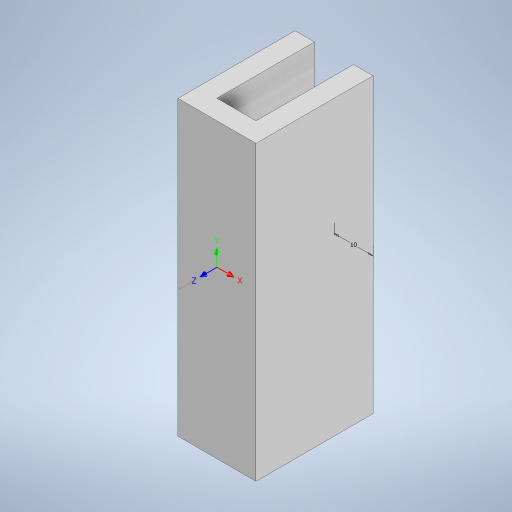
# Autodesk Inventor part: TSU_Middle_Clamp
Saved by Autodesk Inventor 2024 (Build 280153000, 153)
## iProperties
Created: 2024-12-30
Part Number: TSU_Middle_Clamp
Material: Generic
Document SubType Name: Modeling
Designer: mtidd
Density: 1 g/cm^3
Appearance: Default
Author: mtidd
Autodesk Inventor part; units mm, degrees
ref_plane "YZ Plane" through (0, 0, 0) normal (1, 0, 0) x (0, 1, 0)
ref_plane "XZ Plane" through (0, 0, 0) normal (0, 1, 0) x (-1, 0, 0)
ref_plane "XY Plane" through (0, 0, 0) normal (0, 0, 1) x (1, 0, 0)
sketch "Sketch3" plane through (0, 0, 0) normal (0, 1, 0) x (-1, 0, 0)
  line L0 (0, 0) -> (5, 0)
  line L1 (5, 0) -> (-5, 0)
  line L2 (-5, 0) -> (-5, -25)
  line L3 (-5, 0) -> (20, 0) construction
  line L4 (-5, -25) -> (-10, -25)
  line L5 (-10, -25) -> (-10, 5)
  line L6 (-10, 5) -> (0, 5)
  line L7 (0, 5) -> (5, 5)
  line L8 (5, 5) -> (5, 0)
  line L9 (5, 0) -> (5, -25)
  line L10 (5, -25) -> (10, -25)
  line L11 (10, -25) -> (10, 5)
  line L12 (10, 5) -> (5, 5)
  dimension "d2" = 5
  dimension "d3" = 10
  dimension "d4" = 0
  dimension "d5" = 25
  dimension "d6" = 90
  dimension "d7" = 5
  dimension "d8" = 30
  dimension "d9" = 5
  constraints: 26 end point, 7 perpendicular, 5 point on line, 2 horizontal, 1 collinear, 1 vertical
  measures "d2" distance of L0.start L0.end
  measures "d3" distance of L0.end L1.end
  measures "d4" distance between parallel lines of L1 L0
  measures "d5" distance of L1.end L2.end
  measures "d6" angle of L2 L3
  measures "d7" distance of L2.end L4.end
  measures "d8" distance of L4.end L5.end
  measures "d9" distance of L9.end L10.end
extrude "Extrusion1" add sketch "Sketch3" along normal mid plane 75
sketch "Sketch4" plane through (-5, 37.5, -25) normal (0, 0, -1) x (-1, 0, 0)
  line L0 (-5, -37.5) -> (5, -37.5) construction
  line L1 (5, -75) -> (5, 0) construction
  line L2 (-5, -37.5) -> (-15, -37.5) construction
  dimension "d12" = 10
  constraints: 4 end point, 1 midpoint, 1 point on line
  measures "d12" distance of L0.start L2.end
sketch "Sketch6" plane through (-5, -37.5, -25) normal (1, 0, 0) x (0, 0, -1)
  point P0 (-25, 37.5)
body "Solid1"
